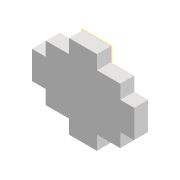
# Autodesk Inventor part: onderkantBovenkant knoppendoosje
Saved by Autodesk Inventor 2020.3 (Build 243373000, 373)
## iProperties
Created: 2020-12-08
Part Number: onderkantBovenkant knoppendoosje
Material: Wood (Birch)
Document SubType Name: Sheet Metal
Designer: Svend
Density: 0.55 g/cm^3
Sheet Metal Rule: Default
Appearance: Birch - Natural Polished
Author: Svend
Autodesk Inventor part; units mm, degrees
ref_plane "YZ Plane" through (0, 0, 0) normal (1, 0, 0) x (0, 1, 0)
ref_plane "XZ Plane" through (0, 0, 0) normal (0, 1, 0) x (-1, 0, 0)
ref_plane "XY Plane" through (0, 0, 0) normal (0, 0, 1) x (1, 0, 0)
ref_plane "Work Plane1" through (0, 30, 0) normal (0, 0, 1) x (1, 0, 0)
sketch "Sketch1" plane through (0, 30, 0) normal (0, 0, 1) x (1, 0, 0)
  line L0 (0, 6) -> (12, 6) projected
  line L1 (0, 0) -> (0, 6) projected
  line L2 (12, 0) -> (0, 0) projected
  line L3 (12, 0) -> (12, 6) projected
  line L4 (28, -6) -> (28, -18) projected
  line L5 (22, -6) -> (28, -6) projected
  line L6 (22, -18) -> (22, -6) projected
  line L7 (22, -18) -> (28, -18) projected
  line L8 (0, -24) -> (12, -24) projected
  line L9 (0, -30) -> (0, -24) projected
  line L10 (12, -30) -> (0, -30) projected
  line L11 (12, -30) -> (12, -24) projected
  line L12 (-10, -6) -> (-10, -18) projected
  line L13 (-16, -6) -> (-10, -6) projected
  line L14 (-16, -18) -> (-16, -6) projected
  line L15 (-16, -18) -> (-10, -18) projected
  line L16 (-10, 0) -> (0, 0) projected
  line L17 (12, 0) -> (22, 0) projected
  line L18 (22, 6) -> (22, -6) projected
  line L19 (22, -18) -> (22, -30) projected
  line L20 (12, -24) -> (22, -24) projected
  line L21 (0, -24) -> (-10, -24) projected
  line L22 (-10, -30) -> (-10, -18) projected
  line L23 (-10, -6) -> (-10, 6) projected
extrude "Extrusion1" add sketch "Sketch1" along normal blind 6
equation "\"BendRadius\" = Thickness"
equation "\"BendReliefWidth\" = Thickness"
equation "\"BendReliefDepth\" = 0.5 * Thickness"
equation "\"CornerReliefSize\" = 4 * Thickness"
equation "\"MinimumRemnant\" = 2 * Thickness"
equation "\"TransitionRadius\" = BendRadius"
equation "\"JacobiRadiusSize\" = Thickness"
equation "\"GapSize\" = Thickness"
equation "\"Thickness\" = 0.5"
body "Solid1"
